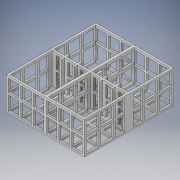
# Autodesk Inventor part: 4 Tape Measures Holder
Saved by Autodesk Inventor 2019 (Build 230136000, 136)
## iProperties
Created: 2018-12-28
Part Number: 4 Tape Measures Holder
Material: Generic
Document SubType Name: Modeling
Designer: ashle
Density: 1 g/cm^3
Appearance: Default
Author: ashle
Autodesk Inventor part; units mm, degrees
ref_plane "YZ Plane" through (0, 0, 0) normal (1, 0, 0) x (0, 1, 0)
ref_plane "XZ Plane" through (0, 0, 0) normal (0, 1, 0) x (-1, 0, 0)
ref_plane "XY Plane" through (0, 0, 0) normal (0, 0, 1) x (1, 0, 0)
sketch "Sketch1" plane through (0, 0, 0) normal (0, 1, 0) x (-1, 0, 0)
  line L0 (2743.2, 3327.4) -> (-2743.2, 3327.4)
  line L1 (-2743.2, 3327.4) -> (-2743.2, 3175)
  line L2 (-2743.2, 3175) -> (2743.2, 3175)
  line L3 (2743.2, 3175) -> (2743.2, 3327.4)
  line L4 (0, 5131.2687) -> (0, -6149.1862) construction
  line L5 (2743.2, 4620.3571) -> (2743.2, -4424.6448) construction
  line L6 (-2743.2, 4620.3571) -> (-2743.2, -5005.5165) construction
  line L7 (-3643.9458, -3175) -> (3603.587, -3175) construction
  line L8 (3452.6337, 3175) -> (-4564.2023, 3175) construction
  line L9 (-2743.2, 2243.6667) -> (-2743.2, 2091.2667)
  line L10 (2743.2, 2243.6667) -> (-2743.2, 2243.6667)
  line L11 (-2743.2, 2091.2667) -> (2743.2, 2091.2667)
  line L12 (2743.2, 2091.2667) -> (2743.2, 2243.6667)
  line L13 (-2743.2, 1159.9333) -> (-2743.2, 1007.5333)
  line L14 (2743.2, 1159.9333) -> (-2743.2, 1159.9333)
  line L15 (-2743.2, 1007.5333) -> (2743.2, 1007.5333)
  line L16 (2743.2, 1007.5333) -> (2743.2, 1159.9333)
  line L17 (-2743.2, -317.5) -> (2743.2, -317.5)
  line L18 (2743.2, -317.5) -> (2743.2, 317.5)
  line L19 (2743.2, 317.5) -> (-2743.2, 317.5)
  line L20 (-2743.2, 317.5) -> (-2743.2, -317.5)
  line L21 (-2743.2, -317.5) -> (2743.2, 317.5) construction
  line L22 (2743.2, -317.5) -> (-2743.2, 317.5) construction
  line L23 (-101.6, -3327.4) -> (101.6, -3327.4)
  line L24 (101.6, -3327.4) -> (101.6, 3327.4)
  line L25 (101.6, 3327.4) -> (-101.6, 3327.4)
  line L26 (-101.6, 3327.4) -> (-101.6, -3327.4)
  line L27 (-101.6, -3327.4) -> (101.6, 3327.4) construction
  line L28 (101.6, -3327.4) -> (-101.6, 3327.4) construction
  line L29 (3750.9383, 0) -> (-5642.9813, 0) construction
  line L30 (2743.2, -3327.4) -> (-2743.2, -3327.4)
  line L31 (-2743.2, -3327.4) -> (-2743.2, -3175)
  line L32 (-2743.2, -3175) -> (2743.2, -3175)
  line L33 (2743.2, -3175) -> (2743.2, -3327.4)
  line L34 (-2743.2, -2243.6667) -> (-2743.2, -2091.2667)
  line L35 (2743.2, -2243.6667) -> (-2743.2, -2243.6667)
  line L36 (-2743.2, -2091.2667) -> (2743.2, -2091.2667)
  line L37 (2743.2, -2091.2667) -> (2743.2, -2243.6667)
  line L38 (-2743.2, -1159.9333) -> (-2743.2, -1007.5333)
  line L39 (2743.2, -1159.9333) -> (-2743.2, -1159.9333)
  line L40 (-2743.2, -1007.5333) -> (2743.2, -1007.5333)
  line L41 (2743.2, -1007.5333) -> (2743.2, -1159.9333)
  line L42 (2895.6, 3327.4) -> (2743.2, 3327.4)
  line L43 (2743.2, 3327.4) -> (2743.2, -3327.4)
  line L44 (2743.2, -3327.4) -> (2895.6, -3327.4)
  line L45 (2895.6, -3327.4) -> (2895.6, 3327.4)
  line L46 (1803.4, 3327.4) -> (1803.4, -3327.4)
  line L47 (1955.8, -3327.4) -> (1955.8, 3327.4)
  line L48 (1955.8, 3327.4) -> (1803.4, 3327.4)
  line L49 (1803.4, -3327.4) -> (1955.8, -3327.4)
  line L50 (863.6, 3327.4) -> (863.6, -3327.4)
  line L51 (1016, -3327.4) -> (1016, 3327.4)
  line L52 (1016, 3327.4) -> (863.6, 3327.4)
  line L53 (863.6, -3327.4) -> (1016, -3327.4)
  line L54 (-2895.6, 3327.4) -> (-2743.2, 3327.4)
  line L55 (-2743.2, 3327.4) -> (-2743.2, -3327.4)
  line L56 (-2743.2, -3327.4) -> (-2895.6, -3327.4)
  line L57 (-2895.6, -3327.4) -> (-2895.6, 3327.4)
  line L58 (-1803.4, 3327.4) -> (-1803.4, -3327.4)
  line L59 (-1955.8, -3327.4) -> (-1955.8, 3327.4)
  line L60 (-1955.8, 3327.4) -> (-1803.4, 3327.4)
  line L61 (-1803.4, -3327.4) -> (-1955.8, -3327.4)
  line L62 (-863.6, 3327.4) -> (-863.6, -3327.4)
  line L63 (-1016, -3327.4) -> (-1016, 3327.4)
  line L64 (-1016, 3327.4) -> (-863.6, 3327.4)
  line L65 (-863.6, -3327.4) -> (-1016, -3327.4)
  point P0 (0, 0)
  point P1 (-1803.4, 3327.4)
  dimension "d0" = 5486.4
  dimension "d1" = 152.4
  dimension "d5" = 2743.2
  dimension "d6" = 3175
  dimension "d7" = 6350
  dimension "d10" = 1083.7333
  dimension "d15" = 635
  dimension "d16" = 203.2
  dimension "d19" = 2015.0667
  dimension "d20" = 2015.0667
  dimension "d21" = 152.4
  dimension "d24" = 939.8
  dimension "d29" = 1727.2
  dimension "d30" = 1727.2
  dimension "d32" = 939.8
  dimension "d33" = 1083.7333
  dimension "d36" = 152.4
  dimension "d37" = 152.4
  constraints: 132 end point, 28 symmetric about line, 8 collinear, 8 horizontal, 8 parallel, 4 midpoint, 4 perpendicular, 4 vertical, 36 other
  measures "d0" distance of L0.start L0.end
  measures "d1" distance of L2.end L0.start
  measures "d5" distance from line of point (0, 0) L1
  measures "d6" distance from line of point (0, 0) L2
  measures "d7" distance between parallel lines of L7 L8
  measures "d10" distance of L0.end L9.start
  measures "d15" distance between parallel lines of L17 L19
  measures "d16" distance between parallel lines of L26 L24
  measures "d19" distance between parallel lines of L14 L2
  measures "d20" distance between parallel lines of L40 L15
  measures "d21" distance of L42.start L42.end
  measures "d24" distance of L42.end L46.start
  measures "d29" distance between parallel lines of L43 L51
  measures "d30" distance between parallel lines of L62 L50
  measures "d32" distance between parallel lines of L58 L62
  measures "d33" distance between parallel lines of L40 L36
  measures "d36" distance between parallel lines of L35 L36
  measures "d37" distance between parallel lines of L59 L58
extrude "Extrusion1" add sketch "Sketch1" along normal blind 127 contours L3 L2 L47 L0 | L42 L45 L44 L33 L43 L37 L41 L18 L16 L12 L3 | L47 L2 L46 L0 | L46 L2 L51 L0 | L47 L10 L46 L2 | L12 L11 L47 L10 | L51 L2 L50 L0 | L47 L11 L46 L10 | L30 L47 L32 L33 | L50 L2 L24 L0 | L51 L10 L50 L2 | L46 L11 L51 L10 | L47 L14 L46 L11 | L16 L15 L47 L14 | L30 L46 L32 L47 | L24 L2 L26 L0 | L51 L11 L50 L10 | L47 L15 L46 L14 | L30 L51 L32 L46 | L32 L46 L35 L47 | L35 L47 L36 L37 | L26 L2 L62 L0 | L24 L10 L26 L2 | L50 L11 L24 L10 | L51 L14 L50 L11 | L46 L15 L51 L14 | L47 L19 L46 L15 | L18 L17 L47 L19 | L30 L50 L32 L51 | L35 L46 L36 L47 | L62 L2 L63 L0 | L24 L11 L26 L10 | L51 L15 L50 L14 | L47 L17 L46 L19 | L30 L24 L32 L50 | L32 L50 L35 L51 | L35 L51 L36 L46 | L36 L46 L39 L47 | L39 L47 L40 L41 | L63 L2 L58 L0 | L62 L10 L63 L2 | L26 L11 L62 L10 | L24 L14 L26 L11 | L50 L15 L24 L14 | L51 L19 L50 L15 | L46 L17 L51 L19 | L47 L40 L46 L17 | L23 L26 L32 L24 | L35 L50 L36 L51 | L39 L46 L40 L47 | L58 L2 L59 L0 | L62 L11 L63 L10 | L24 L15 L26 L14 | L51 L17 L50 L19 | L30 L62 L32 L26 | L32 L26 L35 L24 | L35 L24 L36 L50 | L36 L50 L39 L51 | L39 L51 L40 L46 | L59 L2 L1 L0 | L58 L10 L59 L2 | L63 L11 L58 L10 | L62 L14 L63 L11 | L26 L15 L62 L14 | L24 L19 L26 L15 | L50 L17 L24 L19 | L51 L40 L50 L17 | L30 L63 L32 L62 | L35 L26 L36 L24 | L39 L50 L40 L51 | L1 L55 L9 L13 L20 L38 L34 L31 L56 L57 L54 | L58 L11 L59 L10 | L62 L15 L63 L14 | L24 L17 L26 L19 | L35 L62 L36 L26 | L32 L63 L35 L62 | L30 L58 L32 L63 | L36 L26 L39 L24 | L39 L24 L40 L50 | L59 L11 L9 L10 | L58 L14 L59 L11 | L63 L15 L58 L14 | L62 L19 L63 L15 | L26 L17 L62 L19 | L24 L40 L26 L17 | L35 L63 L36 L62 | L30 L59 L32 L58 | L39 L26 L40 L24 | L58 L15 L59 L14 | L62 L17 L63 L19 | L39 L62 L40 L26 | L36 L63 L39 L62 | L35 L58 L36 L63 | L32 L59 L35 L58 | L30 L31 L32 L59 | L59 L15 L13 L14 | L58 L19 L59 L15 | L63 L17 L58 L19 | L62 L40 L63 L17 | L39 L63 L40 L62 | L35 L59 L36 L58 | L58 L17 L59 L19 | L39 L58 L40 L63 | L36 L59 L39 L58 | L35 L34 L36 L59 | L59 L17 L20 L19 | L58 L40 L59 L17 | L39 L59 L40 L58 | L39 L38 L40 L59
sketch "Sketch3" plane through (0, 127, 0) normal (0, 1, 0) x (1, 0, 0)
  line L0 (-2895.6, -3327.4) -> (2895.6, -3327.4) construction
  line L1 (-2895.6, -3327.4) -> (-2743.2, -3327.4)
  line L2 (-2743.2, -3327.4) -> (-2743.2, -3175)
  line L3 (-2743.2, -3175) -> (-2895.6, -3175)
  line L4 (-2895.6, -3175) -> (-2895.6, -3327.4)
  line L5 (-1955.8, -3175) -> (-2743.2, -3175) construction
  line L6 (-2743.2, -3175) -> (-2743.2, -2243.6667) construction
  line L7 (-2895.6, -2243.6667) -> (-2743.2, -2243.6667)
  line L8 (-2743.2, -2243.6667) -> (-2743.2, -2091.2667)
  line L9 (-2743.2, -2091.2667) -> (-2895.6, -2091.2667)
  line L10 (-2895.6, -2091.2667) -> (-2895.6, -2243.6667)
  line L11 (-2895.6, -1159.9333) -> (-2743.2, -1159.9333)
  line L12 (-2743.2, -1159.9333) -> (-2743.2, -1007.5333)
  line L13 (-2743.2, -1007.5333) -> (-2895.6, -1007.5333)
  line L14 (-2895.6, -1007.5333) -> (-2895.6, -1159.9333)
  line L15 (-2895.6, 1007.5333) -> (-2743.2, 1007.5333)
  line L16 (-2743.2, 1007.5333) -> (-2743.2, 1159.9333)
  line L17 (-2743.2, 1159.9333) -> (-2895.6, 1159.9333)
  line L18 (-2895.6, 1159.9333) -> (-2895.6, 1007.5333)
  line L19 (-2895.6, 3175) -> (-2743.2, 3175)
  line L20 (-2743.2, 3175) -> (-2743.2, 3327.4)
  line L21 (-2743.2, 3327.4) -> (-2895.6, 3327.4)
  line L22 (-2895.6, 3327.4) -> (-2895.6, 3175)
  line L23 (-1955.8, 3175) -> (-1803.4, 3175)
  line L24 (-1803.4, 3175) -> (-1803.4, 3327.4)
  line L25 (-1803.4, 3327.4) -> (-1955.8, 3327.4)
  line L26 (-1955.8, 3327.4) -> (-1955.8, 3175)
  line L27 (-1016, 3175) -> (-863.6, 3175)
  line L28 (-863.6, 3175) -> (-863.6, 3327.4)
  line L29 (-863.6, 3327.4) -> (-1016, 3327.4)
  line L30 (-1016, 3327.4) -> (-1016, 3175)
  line L31 (-101.6, 3327.4) -> (101.6, 3327.4)
  line L32 (101.6, 3327.4) -> (101.6, 3175)
  line L33 (101.6, 3175) -> (-101.6, 3175)
  line L34 (-101.6, 3175) -> (-101.6, 3327.4)
  line L35 (863.6, 3175) -> (1016, 3175)
  line L36 (1016, 3175) -> (1016, 3327.4)
  line L37 (1016, 3327.4) -> (863.6, 3327.4)
  line L38 (863.6, 3327.4) -> (863.6, 3175)
  line L39 (1803.4, 3175) -> (1955.8, 3175)
  line L40 (1955.8, 3175) -> (1955.8, 3327.4)
  line L41 (1955.8, 3327.4) -> (1803.4, 3327.4)
  line L42 (1803.4, 3327.4) -> (1803.4, 3175)
  line L43 (2743.2, 3175) -> (2895.6, 3175)
  line L44 (2895.6, 3175) -> (2895.6, 3327.4)
  line L45 (2895.6, 3327.4) -> (2743.2, 3327.4)
  line L46 (2743.2, 3327.4) -> (2743.2, 3175)
  line L47 (2743.2, 2091.2667) -> (2895.6, 2091.2667)
  line L48 (2895.6, 2091.2667) -> (2895.6, 2243.6667)
  line L49 (2895.6, 2243.6667) -> (2743.2, 2243.6667)
  line L50 (2743.2, 2243.6667) -> (2743.2, 2091.2667)
  line L51 (2895.6, 1159.9333) -> (2743.2, 1159.9333)
  line L52 (2743.2, 1159.9333) -> (2743.2, 1007.5333)
  line L53 (2743.2, 1007.5333) -> (2895.6, 1007.5333)
  line L54 (2895.6, 1007.5333) -> (2895.6, 1159.9333)
  line L55 (2743.2, -317.5) -> (2895.6, -317.5)
  line L56 (2895.6, -317.5) -> (2895.6, 317.5)
  line L57 (2895.6, 317.5) -> (2743.2, 317.5)
  line L58 (2743.2, 317.5) -> (2743.2, -317.5)
  line L59 (2743.2, -1159.9333) -> (2895.6, -1159.9333)
  line L60 (2895.6, -1159.9333) -> (2895.6, -1007.5333)
  line L61 (2895.6, -1007.5333) -> (2743.2, -1007.5333)
  line L62 (2743.2, -1007.5333) -> (2743.2, -1159.9333)
  line L63 (2743.2, -2243.6667) -> (2895.6, -2243.6667)
  line L64 (2895.6, -2243.6667) -> (2895.6, -2091.2667)
  line L65 (2895.6, -2091.2667) -> (2743.2, -2091.2667)
  line L66 (2743.2, -2091.2667) -> (2743.2, -2243.6667)
  line L67 (2743.2, -3327.4) -> (2895.6, -3327.4)
  line L68 (2895.6, -3327.4) -> (2895.6, -3175)
  line L69 (2895.6, -3175) -> (2743.2, -3175)
  line L70 (2743.2, -3175) -> (2743.2, -3327.4)
  line L71 (1803.4, -3327.4) -> (1955.8, -3327.4)
  line L72 (1955.8, -3327.4) -> (1955.8, -3175)
  line L73 (1955.8, -3175) -> (1803.4, -3175)
  line L74 (1803.4, -3175) -> (1803.4, -3327.4)
  line L75 (863.6, -3327.4) -> (1016, -3327.4)
  line L76 (1016, -3327.4) -> (1016, -3175)
  line L77 (1016, -3175) -> (863.6, -3175)
  line L78 (863.6, -3175) -> (863.6, -3327.4)
  line L79 (-101.6, -3327.4) -> (101.6, -3327.4)
  line L80 (101.6, -3327.4) -> (101.6, -3175)
  line L81 (101.6, -3175) -> (-101.6, -3175)
  line L82 (-101.6, -3175) -> (-101.6, -3327.4)
  line L83 (-1016, -3327.4) -> (-863.6, -3327.4)
  line L84 (-863.6, -3327.4) -> (-863.6, -3175)
  line L85 (-863.6, -3175) -> (-1016, -3175)
  line L86 (-1016, -3175) -> (-1016, -3327.4)
  line L87 (-1955.8, -3327.4) -> (-1803.4, -3327.4)
  line L88 (-1803.4, -3327.4) -> (-1803.4, -3175)
  line L89 (-1803.4, -3175) -> (-1955.8, -3175)
  line L90 (-1955.8, -3175) -> (-1955.8, -3327.4)
  line L91 (-1955.8, -317.5) -> (-1803.4, -317.5)
  line L92 (-1803.4, -317.5) -> (-1803.4, 317.5)
  line L93 (-1803.4, 317.5) -> (-1955.8, 317.5)
  line L94 (-1955.8, 317.5) -> (-1955.8, -317.5)
  line L95 (-2895.6, -317.5) -> (-2743.2, -317.5)
  line L96 (-2743.2, -317.5) -> (-2743.2, 317.5)
  line L97 (-2743.2, 317.5) -> (-2895.6, 317.5)
  line L98 (-2895.6, 317.5) -> (-2895.6, -317.5)
  line L99 (-1016, -317.5) -> (-863.6, -317.5)
  line L100 (-863.6, -317.5) -> (-863.6, 317.5)
  line L101 (-863.6, 317.5) -> (-1016, 317.5)
  line L102 (-1016, 317.5) -> (-1016, -317.5)
  line L103 (-101.6, -317.5) -> (101.6, -317.5)
  line L104 (101.6, -317.5) -> (101.6, 317.5)
  line L105 (101.6, 317.5) -> (-101.6, 317.5)
  line L106 (-101.6, 317.5) -> (-101.6, -317.5)
  line L107 (863.6, -317.5) -> (1016, -317.5)
  line L108 (1016, -317.5) -> (1016, 317.5)
  line L109 (1016, 317.5) -> (863.6, 317.5)
  line L110 (863.6, 317.5) -> (863.6, -317.5)
  line L111 (1803.4, -317.5) -> (1955.8, -317.5)
  line L112 (1955.8, -317.5) -> (1955.8, 317.5)
  line L113 (1955.8, 317.5) -> (1803.4, 317.5)
  line L114 (1803.4, 317.5) -> (1803.4, -317.5)
  line L115 (-2743.2, -2243.6667) -> (-1955.8, -2243.6667) construction
  line L116 (-1955.8, -2091.2667) -> (-2743.2, -2091.2667) construction
  line L117 (-2743.2, -2091.2667) -> (-2743.2, -1159.9333) construction
  line L118 (-2743.2, -1159.9333) -> (-1955.8, -1159.9333) construction
  line L119 (-1955.8, -1007.5333) -> (-2743.2, -1007.5333) construction
  line L120 (-2743.2, -1007.5333) -> (-2743.2, -317.5) construction
  line L121 (-2743.2, -317.5) -> (-1955.8, -317.5) construction
  line L122 (-1955.8, 317.5) -> (-2743.2, 317.5) construction
  line L123 (-2743.2, 317.5) -> (-2743.2, 1007.5333) construction
  line L124 (-2743.2, 1007.5333) -> (-1955.8, 1007.5333) construction
  line L125 (-1955.8, 1159.9333) -> (-2743.2, 1159.9333) construction
  line L126 (-2743.2, 3175) -> (-1955.8, 3175) construction
  line L127 (2895.6, 3327.4) -> (-2895.6, 3327.4) construction
  line L128 (-1955.8, 3175) -> (-1955.8, 2243.6667) construction
  line L129 (-1803.4, 2243.6667) -> (-1803.4, 3175) construction
  line L130 (-1016, 3175) -> (-1016, 2243.6667) construction
  line L131 (-863.6, 2243.6667) -> (-863.6, 3175) construction
  line L132 (-101.6, 3175) -> (-101.6, 2243.6667) construction
  line L133 (101.6, 2243.6667) -> (101.6, 3175) construction
  line L134 (863.6, 3175) -> (863.6, 2243.6667) construction
  line L135 (1016, 3175) -> (1803.4, 3175) construction
  line L136 (1016, 2243.6667) -> (1016, 3175) construction
  line L137 (1955.8, 2243.6667) -> (1955.8, 3175) construction
  line L138 (1803.4, 3175) -> (1803.4, 2243.6667) construction
  line L139 (2743.2, 3175) -> (2743.2, 2243.6667) construction
  line L140 (2895.6, -3327.4) -> (2895.6, 3327.4) construction
  line L141 (1955.8, 3175) -> (2743.2, 3175) construction
  line L142 (2743.2, 2243.6667) -> (1955.8, 2243.6667) construction
  line L143 (1955.8, 2091.2667) -> (2743.2, 2091.2667) construction
  line L144 (2743.2, 1159.9333) -> (1955.8, 1159.9333) construction
  line L145 (1955.8, 1007.5333) -> (2743.2, 1007.5333) construction
  line L146 (2743.2, 1007.5333) -> (2743.2, 317.5) construction
  line L147 (2743.2, 317.5) -> (1955.8, 317.5) construction
  line L148 (1955.8, -317.5) -> (2743.2, -317.5) construction
  line L149 (1955.8, -1159.9333) -> (2743.2, -1159.9333) construction
  line L150 (2743.2, -1007.5333) -> (1955.8, -1007.5333) construction
  line L151 (2743.2, -2091.2667) -> (1955.8, -2091.2667) construction
  line L152 (1955.8, -2243.6667) -> (2743.2, -2243.6667) construction
  line L153 (2743.2, -3175) -> (1955.8, -3175) construction
  line L154 (2743.2, -2243.6667) -> (2743.2, -3175) construction
  line L155 (1955.8, -3175) -> (1955.8, -2243.6667) construction
  line L156 (1803.4, -2243.6667) -> (1803.4, -3175) construction
  line L157 (1016, -3175) -> (1016, -2243.6667) construction
  line L158 (863.6, -2243.6667) -> (863.6, -3175) construction
  line L159 (101.6, -3175) -> (101.6, -2243.6667) construction
  line L160 (-101.6, -2243.6667) -> (-101.6, -3175) construction
  line L161 (-863.6, -3175) -> (-863.6, -2243.6667) construction
  line L162 (-1016, -2243.6667) -> (-1016, -3175) construction
  line L163 (-1016, -3175) -> (-1803.4, -3175) construction
  line L164 (-1955.8, -2243.6667) -> (-1955.8, -3175) construction
  line L165 (-1803.4, -3175) -> (-1803.4, -2243.6667) construction
  line L166 (-1955.8, -317.5) -> (-1955.8, -1007.5333) construction
  line L167 (-1803.4, -317.5) -> (-1016, -317.5) construction
  line L168 (-1803.4, 317.5) -> (-1803.4, 1007.5333) construction
  line L169 (-863.6, 317.5) -> (-863.6, 1007.5333) construction
  line L170 (863.6, 317.5) -> (101.6, 317.5) construction
  line L171 (863.6, 1007.5333) -> (863.6, 317.5) construction
  line L172 (1016, 317.5) -> (1016, 1007.5333) construction
  line L173 (-1562.1, 76.2) -> (-2197.1, 76.2)
  line L174 (-2197.1, 76.2) -> (-2197.1, -76.2)
  line L175 (-2197.1, -76.2) -> (-1562.1, -76.2)
  line L176 (-1562.1, -76.2) -> (-1562.1, 76.2)
  line L177 (-1562.1, 76.2) -> (-2197.1, -76.2) construction
  line L178 (-2197.1, 76.2) -> (-1562.1, -76.2) construction
  line L179 (-2957.608, 0) -> (3704.6319, 0) construction
  line L180 (-2895.6, -76.2) -> (-2425.7, -76.2)
  line L181 (-2425.7, -76.2) -> (-2425.7, 76.2)
  line L182 (-2425.7, 76.2) -> (-2895.6, 76.2)
  line L183 (-2895.6, 76.2) -> (-2895.6, -76.2)
  line L184 (-622.3, -76.2) -> (-622.3, 76.2)
  line L185 (-622.3, 76.2) -> (-1257.3, 76.2)
  line L186 (-1257.3, -76.2) -> (-622.3, -76.2)
  line L187 (-1257.3, 76.2) -> (-1257.3, -76.2)
  line L188 (-622.3, 76.2) -> (-1257.3, -76.2) construction
  line L189 (-1257.3, 76.2) -> (-622.3, -76.2) construction
  line L190 (317.5, -76.2) -> (317.5, 76.2)
  line L191 (317.5, 76.2) -> (-317.5, 76.2)
  line L192 (-317.5, -76.2) -> (317.5, -76.2)
  line L193 (-317.5, 76.2) -> (-317.5, -76.2)
  line L194 (317.5, 76.2) -> (-317.5, -76.2) construction
  line L195 (-317.5, 76.2) -> (317.5, -76.2) construction
  line L196 (1257.3, -76.2) -> (1257.3, 76.2)
  line L197 (1257.3, 76.2) -> (622.3, 76.2)
  line L198 (622.3, -76.2) -> (1257.3, -76.2)
  line L199 (622.3, 76.2) -> (622.3, -76.2)
  line L200 (1257.3, 76.2) -> (622.3, -76.2) construction
  line L201 (622.3, 76.2) -> (1257.3, -76.2) construction
  line L202 (2197.1, -76.2) -> (2197.1, 76.2)
  line L203 (2197.1, 76.2) -> (1562.1, 76.2)
  line L204 (1562.1, -76.2) -> (2197.1, -76.2)
  line L205 (1562.1, 76.2) -> (1562.1, -76.2)
  line L206 (2197.1, 76.2) -> (1562.1, -76.2) construction
  line L207 (1562.1, 76.2) -> (2197.1, -76.2) construction
  line L208 (2743.2, -1159.9333) -> (2743.2, -2091.2667) construction
  line L209 (-2895.6, 2091.2667) -> (-2743.2, 2091.2667)
  line L210 (-2743.2, 2091.2667) -> (-2743.2, 2243.6667)
  line L211 (-2743.2, 2243.6667) -> (-2895.6, 2243.6667)
  line L212 (-2895.6, 2243.6667) -> (-2895.6, 2091.2667)
  line L213 (-2895.6, 3327.4) -> (-2895.6, -3327.4) construction
  line L214 (-2743.2, 2091.2667) -> (-1955.8, 2091.2667) construction
  line L215 (-2743.2, 2243.6667) -> (-2743.2, 3175) construction
  line L216 (-1955.8, 2243.6667) -> (-2743.2, 2243.6667) construction
  line L217 (2895.6, 3327.4) -> (2895.6, -3327.4) projected
  line L218 (2895.6, 76.2) -> (2425.7, 76.2)
  line L219 (2425.7, 76.2) -> (2425.7, -76.2)
  line L220 (2425.7, -76.2) -> (2895.6, -76.2)
  line L221 (2895.6, -76.2) -> (2895.6, 76.2)
  line L222 (-101.6, 2091.2667) -> (101.6, 2091.2667)
  line L223 (101.6, 2091.2667) -> (101.6, 2243.6667)
  line L224 (101.6, 2243.6667) -> (-101.6, 2243.6667)
  line L225 (-101.6, 2243.6667) -> (-101.6, 2091.2667)
  line L226 (-101.6, 2091.2667) -> (101.6, 2243.6667) construction
  line L227 (101.6, 2091.2667) -> (-101.6, 2243.6667) construction
  line L228 (863.6, 2243.6667) -> (101.6, 2243.6667) construction
  line L229 (101.6, 2091.2667) -> (863.6, 2091.2667) construction
  line L230 (-101.6, 1007.5333) -> (101.6, 1007.5333)
  line L231 (101.6, 1007.5333) -> (101.6, 1159.9333)
  line L232 (101.6, 1159.9333) -> (-101.6, 1159.9333)
  line L233 (-101.6, 1159.9333) -> (-101.6, 1007.5333)
  line L234 (-101.6, 1007.5333) -> (101.6, 1159.9333) construction
  line L235 (101.6, 1007.5333) -> (-101.6, 1159.9333) construction
  line L236 (863.6, 1159.9333) -> (101.6, 1159.9333) construction
  line L237 (101.6, 1007.5333) -> (863.6, 1007.5333) construction
  line L238 (-101.6, -1159.9333) -> (101.6, -1159.9333)
  line L239 (101.6, -1159.9333) -> (101.6, -1007.5333)
  line L240 (101.6, -1007.5333) -> (-101.6, -1007.5333)
  line L241 (-101.6, -1007.5333) -> (-101.6, -1159.9333)
  line L242 (-101.6, -1159.9333) -> (101.6, -1007.5333) construction
  line L243 (101.6, -1159.9333) -> (-101.6, -1007.5333) construction
  line L244 (101.6, -2091.2667) -> (101.6, -1159.9333) construction
  line L245 (-101.6, -1159.9333) -> (-101.6, -2091.2667) construction
  line L246 (101.6, -1159.9333) -> (863.6, -1159.9333) construction
  line L247 (863.6, -1007.5333) -> (101.6, -1007.5333) construction
  line L248 (-101.6, -2243.6667) -> (101.6, -2243.6667)
  line L249 (101.6, -2243.6667) -> (101.6, -2091.2667)
  line L250 (101.6, -2091.2667) -> (-101.6, -2091.2667)
  line L251 (-101.6, -2091.2667) -> (-101.6, -2243.6667)
  line L252 (-101.6, -2243.6667) -> (101.6, -2091.2667) construction
  line L253 (101.6, -2243.6667) -> (-101.6, -2091.2667) construction
  line L254 (863.6, -2091.2667) -> (101.6, -2091.2667) construction
  line L255 (-863.6, -2243.6667) -> (-101.6, -2243.6667) construction
  point P0 (0, 0)
  point P1 (-1879.6, 0)
  point P2 (-1879.6, 0)
  point P3 (-939.8, 0)
  point P4 (-939.8, 0)
  point P5 (0, 0)
  point P6 (0, 0)
  point P7 (939.8, 0)
  point P8 (939.8, 0)
  point P9 (1879.6, 0)
  point P10 (1879.6, 0)
  point P11 (0, 2167.4667)
  point P12 (0, 1083.7333)
  point P13 (0, -1083.7333)
  point P14 (0, -2167.4667)
  dimension "d38" = 152.4
  dimension "d39" = 152.4
  dimension "d40" = 76.2
  dimension "d41" = 635
  dimension "d42" = 635
  dimension "d43" = 635
  dimension "d44" = 469.9
  dimension "d45" = 76.2
  dimension "d46" = 76.2
  dimension "d47" = 228.6
  dimension "d50" = 939.8
  dimension "d55" = 76.2
  dimension "d56" = 317.5
  dimension "d65" = 469.9
  constraints: 358 end point, 97 collinear, 72 parallel, 39 horizontal, 36 perpendicular, 34 point on line, 19 midpoint, 4 vertical, 51 other
  measures "d38" distance of L91.start L91.end
  measures "d39" distance of L173.end L174.end
  measures "d40" distance from line of point (-1879.6, 0) L94
  measures "d41" distance of L93.end L91.start
  measures "d42" distance of L173.start L173.end
  measures "d43" distance of L95.end L96.end
  measures "d44" distance of L180.start L180.end
  measures "d45" distance between parallel lines of L179 L182
  measures "d46" distance between parallel lines of L179 L180
  measures "d47" distance between parallel lines of L174 L181
  measures "d50" distance of L175.end L184.start
  measures "d55" distance from line of L114 point (1879.6, 0)
  measures "d56" distance from line of L113 point (1879.6, 0)
  measures "d65" distance between parallel lines of L56 L219
extrude "Extrusion2" add sketch "Sketch3" along normal blind 2286
sketch "Sketch4" plane through (-2895.6, 0, 3327.4) normal (0, 0, 1) x (1, 0, 0)
  line L0 (76.2, 3047.8693) -> (76.2, -507.8693) construction
  line L1 (152.4, 127) -> (152.4, 2413) construction
  line L2 (0, 0) -> (0, 2413) construction
  line L3 (152.4, 1193.8) -> (0, 1193.8)
  line L4 (0, 1193.8) -> (0, 1346.2)
  line L5 (0, 1346.2) -> (152.4, 1346.2)
  line L6 (152.4, 1346.2) -> (152.4, 1193.8)
  line L7 (152.4, 1193.8) -> (0, 1346.2) construction
  line L8 (0, 1193.8) -> (152.4, 1346.2) construction
  line L9 (0, 2413) -> (152.4, 2413) projected
  line L10 (152.4, 127) -> (939.8, 127) construction
  line L11 (152.4, 2260.6) -> (0, 2260.6)
  line L12 (0, 2260.6) -> (0, 2413)
  line L13 (0, 2413) -> (152.4, 2413)
  line L14 (152.4, 2413) -> (152.4, 2260.6)
  line L15 (152.4, 2260.6) -> (0, 2413) construction
  line L16 (0, 2260.6) -> (152.4, 2413) construction
  line L17 (2895.6, 2548.3206) -> (2895.6, -330.2) construction
  line L18 (4851.4, 127) -> (5638.8, 127) construction
  line L19 (5638.8, 1193.8) -> (5791.2, 1193.8)
  line L20 (5791.2, 1193.8) -> (5791.2, 1346.2)
  line L21 (5791.2, 1346.2) -> (5638.8, 1346.2)
  line L22 (5638.8, 1346.2) -> (5638.8, 1193.8)
  line L23 (5638.8, 1193.8) -> (5791.2, 1346.2) construction
  line L24 (5791.2, 1193.8) -> (5638.8, 1346.2) construction
  line L25 (5791.2, 2413) -> (5638.8, 2413)
  line L26 (5638.8, 2260.6) -> (5791.2, 2260.6)
  line L27 (5791.2, 2260.6) -> (5791.2, 2413)
  line L28 (5791.2, 2413) -> (5638.8, 2413)
  line L29 (5638.8, 2413) -> (5638.8, 2260.6)
  line L30 (5638.8, 2260.6) -> (5791.2, 2413) construction
  line L31 (5791.2, 2260.6) -> (5638.8, 2413) construction
  line L32 (2794, 127) -> (2794, 2413) construction
  line L33 (2997.2, 1168.4) -> (2794, 1168.4)
  line L34 (2794, 1168.4) -> (2794, 1371.6)
  line L35 (2794, 1371.6) -> (2997.2, 1371.6)
  line L36 (2997.2, 1371.6) -> (2997.2, 1168.4)
  line L37 (2997.2, 1168.4) -> (2794, 1371.6) construction
  line L38 (2794, 1168.4) -> (2997.2, 1371.6) construction
  line L39 (2032, 127) -> (2794, 127) construction
  line L40 (2997.2, 2209.8) -> (2794, 2209.8)
  line L41 (2794, 2209.8) -> (2794, 2413)
  line L42 (2794, 2413) -> (2997.2, 2413)
  line L43 (2997.2, 2413) -> (2997.2, 2209.8)
  line L44 (2997.2, 2209.8) -> (2794, 2413) construction
  line L45 (2794, 2209.8) -> (2997.2, 2413) construction
  line L46 (2794, 2413) -> (2997.2, 2413) projected
  line L47 (2997.2, 127) -> (2997.2, 2413) projected
  point P0 (2895.6, 0)
  point P1 (76.2, 1270)
  point P2 (76.2, 2336.8)
  point P3 (5715, 1270)
  point P4 (5715, 2336.8)
  point P5 (2895.6, 1270)
  point P6 (2895.6, 2311.4)
  dimension "d59" = 152.4
  dimension "d60" = 76.2
  dimension "d61" = 152.4
  dimension "d62" = 2286
  dimension "d63" = 1143
  dimension "d64" = 152.4
  dimension "d67" = 1143
  dimension "d70" = 203.2
  dimension "d71" = 203.2
  dimension "d72" = 1143
  dimension "d73" = 203.2
  constraints: 78 end point, 13 midpoint, 12 symmetric about line, 8 parallel, 5 collinear, 4 horizontal, 4 perpendicular, 4 point on line, 3 vertical
  measures "d59" distance between parallel lines of L1 L2
  measures "d60" distance between parallel lines of L1 L0
  measures "d61" distance between parallel lines of L3 L5
  measures "d62" distance between parallel lines of L9 L10
  measures "d63" distance from line of L10 point (76.2, 1270)
  measures "d64" distance between parallel lines of L13 L11
  measures "d67" distance from line of L18 point (5715, 1270)
  measures "d70" distance between parallel lines of L33 L35
  measures "d71" distance between parallel lines of L36 L34
  measures "d72" distance from line of L39 point (2895.6, 1270)
  measures "d73" distance between parallel lines of L42 L40
extrude "Extrusion3" add sketch "Sketch4" against normal up to surface (6654.8 mm away)
sketch "Sketch5" plane through (-2895.6, 0, -3327.4) normal (-1, 0, 0) x (0, 0, 1)
  line L0 (0, 2413) -> (152.4, 2413)
  line L1 (152.4, 2413) -> (152.4, 2260.6)
  line L2 (152.4, 2260.6) -> (0, 2260.6)
  line L3 (0, 2260.6) -> (0, 2413)
  line L4 (0, 2413) -> (152.4, 2260.6) construction
  line L5 (152.4, 2413) -> (0, 2260.6) construction
  line L6 (0, 2413) -> (6654.8, 2413) construction
  line L7 (0, 0) -> (0, 2413) construction
  line L8 (1083.7333, 2260.6) -> (152.4, 2260.6) construction
  line L9 (152.4, 1346.2) -> (152.4, 2260.6) construction
  line L10 (152.4, 1193.8) -> (0, 1193.8)
  line L11 (0, 1193.8) -> (0, 1346.2)
  line L12 (0, 1346.2) -> (152.4, 1346.2)
  line L13 (152.4, 1346.2) -> (152.4, 1193.8)
  line L14 (152.4, 1193.8) -> (0, 1346.2) construction
  line L15 (0, 1193.8) -> (152.4, 1346.2) construction
  line L16 (1083.7333, 1346.2) -> (152.4, 1346.2) construction
  line L17 (1083.7333, 1193.8) -> (152.4, 1193.8) construction
  line L18 (3403.6, 1193.8) -> (3251.2, 1193.8)
  line L19 (3251.2, 1193.8) -> (3251.2, 1346.2)
  line L20 (3251.2, 1346.2) -> (3403.6, 1346.2)
  line L21 (3403.6, 1346.2) -> (3403.6, 1193.8)
  line L22 (3403.6, 1193.8) -> (3251.2, 1346.2) construction
  line L23 (3251.2, 1193.8) -> (3403.6, 1346.2) construction
  line L24 (3251.2, 127) -> (3251.2, 2413) construction
  line L25 (3009.9, 1346.2) -> (2319.8667, 1346.2) construction
  line L26 (3403.6, 2413) -> (3403.6, 127) construction
  line L27 (3009.9, 1193.8) -> (2319.8667, 1193.8) construction
  line L28 (3251.2, 2260.6) -> (3403.6, 2260.6)
  line L29 (3403.6, 2260.6) -> (3403.6, 2413)
  line L30 (3403.6, 2413) -> (3251.2, 2413)
  line L31 (3251.2, 2413) -> (3251.2, 2260.6)
  line L32 (3251.2, 2260.6) -> (3403.6, 2413) construction
  line L33 (3403.6, 2260.6) -> (3251.2, 2413) construction
  line L34 (4334.9333, 2260.6) -> (3644.9, 2260.6) construction
  line L35 (6654.8, 2260.6) -> (6502.4, 2260.6)
  line L36 (6502.4, 2260.6) -> (6502.4, 2413)
  line L37 (6502.4, 2413) -> (6654.8, 2413)
  line L38 (6654.8, 2413) -> (6654.8, 2260.6)
  line L39 (6654.8, 2260.6) -> (6502.4, 2413) construction
  line L40 (6502.4, 2260.6) -> (6654.8, 2413) construction
  line L41 (6502.4, 1346.2) -> (6502.4, 2260.6) construction
  line L42 (6654.8, 0) -> (6654.8, 2413) construction
  line L43 (6502.4, 2260.6) -> (5571.0667, 2260.6) construction
  line L44 (6654.8, 1193.8) -> (6502.4, 1193.8)
  line L45 (6502.4, 1193.8) -> (6502.4, 1346.2)
  line L46 (6502.4, 1346.2) -> (6654.8, 1346.2)
  line L47 (6654.8, 1346.2) -> (6654.8, 1193.8)
  line L48 (6654.8, 1193.8) -> (6502.4, 1346.2) construction
  line L49 (6502.4, 1193.8) -> (6654.8, 1346.2) construction
  line L50 (6502.4, 1346.2) -> (5571.0667, 1346.2) construction
  line L51 (6502.4, 1193.8) -> (5571.0667, 1193.8) construction
  point P0 (3327.4, 0)
  point P1 (76.2, 2336.8)
  point P2 (76.2, 1270)
  point P3 (3327.4, 1270)
  point P4 (3327.4, 2336.8)
  point P5 (6578.6, 2336.8)
  point P6 (6578.6, 1270)
  constraints: 72 end point, 24 collinear, 12 midpoint, 12 parallel, 6 horizontal, 6 perpendicular
extrude "Extrusion4" add sketch "Sketch5" against normal up to surface (5791.2 mm away)
sketch "Sketch7" plane through (101.6, 127, -76.2) normal (1, 0, 0) x (0, 0, -1)
  circle A0 centre (1007.5333, 2184.4) radius 50.8
  line L0 (1083.7333, 1244.6) -> (1083.7333, 2082.8) construction
  line L1 (931.3333, 1244.6) -> (931.3333, 2082.8) construction
  line L2 (1083.7333, 2082.8) -> (2015.0667, 2082.8) construction
  line L3 (0, 2286) -> (3098.8, 2286) construction
  line L4 (241.3, 2082.8) -> (931.3333, 2082.8) construction
  circle A1 centre (2091.2667, 2184.4) radius 50.8
  line L5 (2167.4667, 1244.6) -> (2167.4667, 2082.8) construction
  circle A2 centre (-2243.6667, 2184.4) radius 50.8
  line L6 (-2319.8667, 1244.6) -> (-2319.8667, 2082.8) construction
  line L7 (-3251.2, 2286) -> (-152.4, 2286) construction
  circle A3 centre (-1159.9333, 2184.4) radius 50.8
  line L8 (-1236.1333, 1244.6) -> (-1236.1333, 2082.8) construction
  circle A4 centre (-2243.6667, 1930.4) radius 50.8
  line L9 (-2167.4667, 1244.6) -> (-2167.4667, 2082.8) construction
  circle A5 centre (-1159.9333, 1930.4) radius 50.8
  circle A6 centre (1007.5333, 1930.4) radius 50.8
  circle A7 centre (2091.2667, 1930.4) radius 50.8
  line L10 (2015.0667, 1244.6) -> (2015.0667, 2082.8) construction
  point P0 (-76.2, -127)
  dimension "d92" = 101.6
  dimension "d93" = 152.4
  dimension "d94" = 76.2
  dimension "d95" = 203.2
  dimension "d96" = 101.6
  dimension "d97" = 76.2
  dimension "d98" = 101.6
  dimension "d99" = 101.6
  dimension "d100" = 76.2
  dimension "d101" = 101.6
  dimension "d102" = 101.6
  dimension "d103" = 76.2
  dimension "d104" = 101.6
  dimension "d105" = 101.6
  dimension "d106" = 101.6
  dimension "d107" = 76.2
  dimension "d110" = 101.6
  dimension "d111" = 254
  dimension "d112" = 76.2
  dimension "d113" = 101.6
  dimension "d114" = 254
  dimension "d115" = 76.2
  dimension "d116" = 101.6
  dimension "d117" = 76.2
  dimension "d118" = 254
  dimension "d119" = 101.6
  dimension "d120" = 76.2
  dimension "d121" = 254
  constraints: 8 centre point
  measures "d92" diameter of A0
  measures "d93" distance between parallel lines of L0 L1
  measures "d94" distance from line of A0.centre L1
  measures "d95" distance between parallel lines of L2 L3
  measures "d96" distance from line of A0.centre L4
  measures "d97" distance from line of A0.centre L0
  measures "d98" distance from line of L3 A0.centre
  measures "d99" diameter of A1
  measures "d100" distance from line of L5 A1.centre
  measures "d101" distance from line of L3 A1.centre
  measures "d102" diameter of A2
  measures "d103" distance from line of A2.centre L6
  measures "d104" distance from line of L7 A2.centre
  measures "d105" diameter of A3
  measures "d106" distance from line of L7 A3.centre
  measures "d107" distance from line of L8 A3.centre
  measures "d110" diameter of A4
  measures "d111" distance of A2.centre A4.centre
  measures "d112" distance from line of L9 A4.centre
  measures "d113" diameter of A5
  measures "d114" distance of A5.centre A3.centre
  measures "d115" distance from line of L8 A5.centre
  measures "d116" diameter of A6
  measures "d117" distance from line of L0 A6.centre
  measures "d118" distance of A0.centre A6.centre
  measures "d119" diameter of A7
  measures "d120" distance from line of L10 A7.centre
  measures "d121" distance of A1.centre A7.centre
extrude "Extrusion5" cut sketch "Sketch7" against normal up to surface (203.2 mm away)
equation "\"d0\" = 2 * d5"
equation "\"d7\" = 2 * d6"
equation "\"d10\" = 0.166667 * d7 + 0.166667 * d1"
equation "\"d20\" = d19"
equation "\"d21\" = d1"
equation "\"d24\" = 0.166667 * d0 + 0.166667 * d21"
equation "\"d30\" = d29"
equation "\"d39\" = d38"
equation "\"d40\" = 0.5 * d38"
equation "\"d42\" = d41"
equation "\"d44\" = 0.5 * d43 + d38"
equation "\"d45\" = 0.5 * d38"
equation "\"d46\" = d45"
equation "\"d50\" = d47 + d42 + d40"
equation "\"d65\" = d44"
equation "\"d60\" = 0.5 * d59"
equation "\"d61\" = d59"
equation "\"d63\" = 0.5 * d62"
equation "\"d64\" = d59"
equation "\"d70\" = d71"
equation "\"d72\" = d63"
equation "\"d73\" = d70"
equation "\"d94\" = 0.5 * d93"
body "Solid1"
